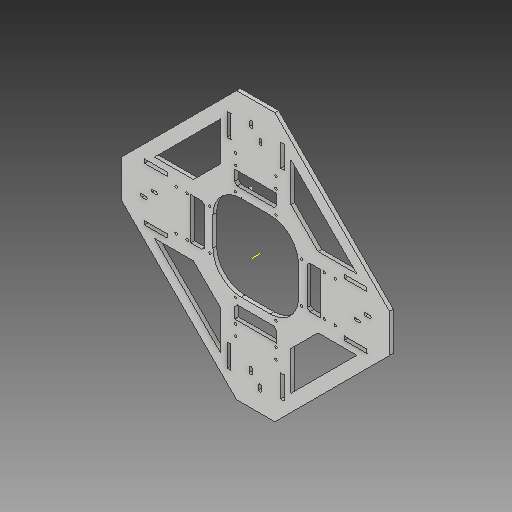
# Autodesk Inventor part: Base Plate
Saved by Autodesk Inventor 2017 (Build 210142000, 142)
## iProperties
Created: 2018-11-23
Part Number: Base Plate
Material: Generic
Document SubType Name: Modeling
Designer: Eric the Great
Density: 1 g/cm^3
Appearance: Default
Author: Eric the Great
Autodesk Inventor part; units mm, degrees
ref_plane "YZ Plane" through (0, 0, 0) normal (1, 0, 0) x (0, 1, 0)
ref_plane "XZ Plane" through (0, 0, 0) normal (0, 1, 0) x (-1, 0, 0)
ref_plane "XY Plane" through (0, 0, 0) normal (0, 0, 1) x (1, 0, 0)
sketch "Sketch1" plane through (0, 0, 0) normal (0, 0, 1) x (1, 0, 0)
  line L0 (79.3342, 54.8946) -> (119.9842, 54.8946)
  line L1 (159.9842, 14.8946) -> (159.9842, -25.7554)
  line L2 (119.9842, -65.7554) -> (79.3342, -65.7554)
  line L3 (39.3342, -25.7554) -> (39.3342, 14.8946)
  line L4 (39.3342, 54.8946) -> (159.9842, -65.7554) construction
  line L5 (159.9842, 54.8946) -> (39.3342, -65.7554) construction
  line L6 (99.6592, 210.0958) -> (315.1854, -5.4304)
  line L7 (315.1854, -5.4304) -> (99.6592, -220.9565)
  line L8 (99.6592, -220.9565) -> (-115.8669, -5.4304)
  line L9 (-115.8669, -5.4304) -> (99.6592, 210.0958)
  line L10 (99.6592, 210.0958) -> (99.6592, -220.9565) construction
  line L11 (315.1854, -5.4304) -> (-115.8669, -5.4304) construction
  arc A0 (39.3342, -25.7554) -> (79.3342, -65.7554) centre (79.3342, -25.7554) ccw
  arc A1 (79.3342, 54.8946) -> (39.3342, 14.8946) centre (79.3342, 14.8946) ccw
  arc A2 (159.9842, 14.8946) -> (119.9842, 54.8946) centre (119.9842, 14.8946) ccw
  arc A3 (119.9842, -65.7554) -> (159.9842, -25.7554) centre (119.9842, -25.7554) ccw
  circle A4 centre (211.7342, 23.0696) radius 1.75 projected
  circle A5 centre (211.7342, -33.9304) radius 1.75 projected
  line L12 (293.5081, -27.1077) -> (293.5081, 16.2469)
  line L13 (195.7506, -101.5218) -> (242.2148, -55.0576)
  line L14 (242.2148, -55.0576) -> (187.4326, -55.0576)
  line L15 (149.2864, -93.2038) -> (149.2864, -147.986)
  line L16 (149.2864, -147.986) -> (195.7506, -101.5218)
  line L17 (168.3595, -74.1307) -> (187.4326, -55.0576)
  line L18 (168.3595, -74.1307) -> (149.2864, -93.2038)
  line L19 (172.0831, 20.9712) -> (172.0831, -31.832)
  line L20 (172.0831, -31.832) -> (176.0974, -34.958)
  line L21 (176.0974, -34.958) -> (191.0974, -34.958)
  line L22 (191.0974, -34.958) -> (191.1331, -34.9121)
  line L23 (191.1331, -34.9121) -> (191.1331, 24.0513)
  line L24 (191.1331, 24.0513) -> (191.0974, 24.0972)
  line L25 (191.0974, 24.0972) -> (176.0974, 24.0972)
  line L26 (176.0974, 24.0972) -> (172.0831, 20.9712)
  line L27 (50.032, -147.986) -> (50.032, -93.2038)
  line L28 (3.5678, -101.5218) -> (50.032, -147.986)
  line L29 (30.9589, -74.1307) -> (50.032, -93.2038)
  line L30 (30.9589, -74.1307) -> (11.8858, -55.0576)
  line L31 (-42.8964, -55.0576) -> (3.5678, -101.5218)
  line L32 (11.8858, -55.0576) -> (-42.8964, -55.0576)
  line L33 (77.9819, -199.2793) -> (121.3365, -199.2793)
  line L34 (126.0608, -77.8543) -> (73.2576, -77.8543)
  line L35 (70.1316, -81.8686) -> (70.1316, -96.8686)
  line L36 (70.1316, -96.8686) -> (70.1775, -96.9043)
  line L37 (129.1868, -81.8686) -> (126.0608, -77.8543)
  line L38 (129.1868, -96.8686) -> (129.1868, -81.8686)
  line L39 (70.1775, -96.9043) -> (129.1409, -96.9043)
  line L40 (129.1409, -96.9043) -> (129.1868, -96.8686)
  line L41 (73.2576, -77.8543) -> (70.1316, -81.8686)
  line L42 (-42.8964, 44.1968) -> (11.8858, 44.1968)
  line L43 (3.5678, 90.661) -> (-42.8964, 44.1968)
  line L44 (30.9589, 63.2699) -> (11.8858, 44.1968)
  line L45 (30.9589, 63.2699) -> (50.032, 82.343)
  line L46 (50.032, 137.1252) -> (3.5678, 90.661)
  line L47 (50.032, 82.343) -> (50.032, 137.1252)
  line L48 (-94.1897, 16.2469) -> (-94.1897, -27.1077)
  line L49 (27.2353, -31.832) -> (27.2353, 20.9712)
  line L50 (23.221, 24.0972) -> (8.221, 24.0972)
  line L51 (8.221, 24.0972) -> (8.1853, 24.0513)
  line L52 (23.221, -34.958) -> (27.2353, -31.832)
  line L53 (8.221, -34.958) -> (23.221, -34.958)
  line L54 (8.1853, 24.0513) -> (8.1853, -34.9121)
  line L55 (8.1853, -34.9121) -> (8.221, -34.958)
  line L56 (27.2353, 20.9712) -> (23.221, 24.0972)
  line L57 (149.2864, 137.1252) -> (149.2864, 82.343)
  line L58 (195.7506, 90.661) -> (149.2864, 137.1252)
  line L59 (168.3595, 63.2699) -> (149.2864, 82.343)
  line L60 (168.3595, 63.2699) -> (187.4326, 44.1968)
  line L61 (242.2148, 44.1968) -> (195.7506, 90.661)
  line L62 (187.4326, 44.1968) -> (242.2148, 44.1968)
  line L63 (121.3365, 188.4185) -> (77.9819, 188.4185)
  line L64 (73.2576, 66.9935) -> (126.0608, 66.9935)
  line L65 (129.1868, 71.0078) -> (129.1868, 86.0078)
  line L66 (129.1868, 86.0078) -> (129.1409, 86.0435)
  line L67 (70.1316, 71.0078) -> (73.2576, 66.9935)
  line L68 (70.1316, 86.0078) -> (70.1316, 71.0078)
  line L69 (129.1409, 86.0435) -> (70.1775, 86.0435)
  line L70 (70.1775, 86.0435) -> (70.1316, 86.0078)
  line L71 (126.0608, 66.9935) -> (129.1868, 71.0078)
  circle A6 centre (128.1592, -101.9862) radius 1.75 projected
  circle A7 centre (71.1592, -101.9862) radius 1.75 projected
  circle A8 centre (71.1592, -117.5054) radius 1.75 projected
  circle A9 centre (128.1592, -117.5054) radius 1.75 projected
  line L72 (95.4092, -166.1418) -> (95.4092, -160.1418) projected
  arc A10 (95.4092, -160.1418) -> (91.4092, -160.1418) centre (93.4092, -160.1418) ccw projected
  arc A11 (91.4092, -166.1418) -> (95.4092, -166.1418) centre (93.4092, -166.1418) ccw projected
  line L73 (103.9092, -145.6418) -> (103.9092, -151.6418) projected
  arc A12 (103.9092, -151.6418) -> (107.9092, -151.6418) centre (105.9092, -151.6418) ccw projected
  line L74 (107.9092, -151.6418) -> (107.9092, -145.6418) projected
  arc A13 (107.9092, -145.6418) -> (103.9092, -145.6418) centre (105.9092, -145.6418) ccw projected
  line L75 (90.8763, -145.4109) -> (90.8763, -151.4109) projected
  line L76 (94.8763, -151.4109) -> (94.8763, -145.4109) projected
  arc A14 (90.8763, -151.4109) -> (94.8763, -151.4109) centre (92.8763, -151.4109) ccw projected
  arc A15 (94.8763, -145.4109) -> (90.8763, -145.4109) centre (92.8763, -145.4109) ccw projected
  arc A16 (107.9092, -160.1418) -> (103.9092, -160.1418) centre (105.9092, -160.1418) ccw projected
  line L77 (103.9092, -160.1418) -> (103.9092, -166.1418) projected
  arc A17 (103.9092, -166.1418) -> (107.9092, -166.1418) centre (105.9092, -166.1418) ccw projected
  line L78 (107.9092, -166.1418) -> (107.9092, -160.1418) projected
  circle A18 centre (128.1592, -70.0054) radius 1.75 projected
  circle A19 centre (71.1592, -70.0054) radius 1.75 projected
  line L79 (139.9592, -130.3297) -> (134.6592, -130.3297) projected
  line L80 (139.9592, -162.0797) -> (134.6592, -162.0797) projected
  line L81 (139.9592, -162.0797) -> (139.9592, -130.3297) projected
  line L82 (134.6592, -130.3297) -> (134.6592, -162.0797) projected
  line L83 (64.6592, -130.3297) -> (59.3592, -130.3297) projected
  line L84 (59.3592, -130.3297) -> (59.3592, -162.0797) projected
  line L85 (64.6592, -162.0797) -> (64.6592, -130.3297) projected
  line L86 (64.6592, -162.0797) -> (59.3592, -162.0797) projected
  line L87 (139.9592, -130.3297) -> (134.6592, -130.3297)
  line L88 (134.6592, -130.3297) -> (134.6592, -162.0797)
  line L89 (134.6592, -162.0797) -> (139.9592, -162.0797)
  line L90 (139.9592, -162.0797) -> (139.9592, -130.3297)
  line L91 (64.6592, -130.3297) -> (59.3592, -130.3297)
  line L92 (59.3592, -130.3297) -> (59.3592, -162.0797)
  line L93 (59.3592, -162.0797) -> (64.6592, -162.0797)
  line L94 (64.6592, -162.0797) -> (64.6592, -130.3297)
  circle A20 centre (128.1592, -70.0054) radius 1.75
  circle A21 centre (71.1592, -70.0054) radius 1.75
  circle A22 centre (71.1592, -101.9862) radius 1.75
  circle A23 centre (71.1592, -117.5054) radius 1.75
  circle A24 centre (128.1592, -117.5054) radius 1.75
  line L95 (92.8763, -151.4109) -> (92.8763, -145.4109) construction
  line L96 (94.4027, -151.4109) -> (94.4027, -145.4109)
  line L97 (91.35, -145.4109) -> (91.35, -151.4109)
  arc A25 (91.35, -151.4109) -> (94.4027, -151.4109) centre (92.8763, -151.4109) ccw
  arc A26 (94.4027, -145.4109) -> (91.35, -145.4109) centre (92.8763, -145.4109) ccw
  line L98 (105.9092, -166.1418) -> (105.9092, -160.1418) construction
  line L99 (107.9092, -166.1418) -> (107.9092, -160.1418)
  line L100 (103.9092, -160.1418) -> (103.9092, -166.1418)
  arc A27 (103.9092, -166.1418) -> (107.9092, -166.1418) centre (105.9092, -166.1418) ccw
  arc A28 (107.9092, -160.1418) -> (103.9092, -160.1418) centre (105.9092, -160.1418) ccw
  circle A29 centre (128.1592, -101.9862) radius 1.75
  circle A30 centre (164.2342, 23.0696) radius 1.75
  circle A31 centre (164.2342, -33.9304) radius 1.75
  circle A32 centre (196.215, 23.0696) radius 1.75
  circle A33 centre (211.7342, 23.0696) radius 1.75
  circle A34 centre (196.215, -33.9304) radius 1.75
  circle A35 centre (211.7342, -33.9304) radius 1.75
  circle A36 centre (71.1592, 59.1446) radius 1.75
  circle A37 centre (128.1592, 59.1446) radius 1.75
  circle A38 centre (71.1592, 91.1254) radius 1.75
  circle A39 centre (71.1592, 106.6446) radius 1.75
  circle A40 centre (128.1592, 91.1254) radius 1.75
  circle A41 centre (128.1592, 106.6446) radius 1.75
  circle A42 centre (35.0842, -33.9304) radius 1.75
  circle A43 centre (35.0842, 23.0696) radius 1.75
  circle A44 centre (3.1034, -33.9304) radius 1.75
  circle A45 centre (-12.4158, -33.9304) radius 1.75
  circle A46 centre (3.1034, 23.0696) radius 1.75
  circle A47 centre (-12.4158, 23.0696) radius 1.75
  line L101 (256.3086, -45.7304) -> (256.3086, -40.4304)
  line L102 (256.3086, -40.4304) -> (224.5586, -40.4304)
  line L103 (224.5586, -40.4304) -> (224.5586, -45.7304)
  line L104 (224.5586, -45.7304) -> (256.3086, -45.7304)
  line L105 (224.5586, 34.8696) -> (224.5586, 29.5696)
  line L106 (256.3086, 29.5696) -> (256.3086, 34.8696)
  line L107 (224.5586, 29.5696) -> (256.3086, 29.5696)
  line L108 (256.3086, 34.8696) -> (224.5586, 34.8696)
  line L109 (139.9592, 151.219) -> (134.6592, 151.219)
  line L110 (134.6592, 151.219) -> (134.6592, 119.469)
  line L111 (134.6592, 119.469) -> (139.9592, 119.469)
  line L112 (139.9592, 119.469) -> (139.9592, 151.219)
  line L113 (59.3592, 119.469) -> (64.6592, 119.469)
  line L114 (64.6592, 151.219) -> (59.3592, 151.219)
  line L115 (64.6592, 119.469) -> (64.6592, 151.219)
  line L116 (59.3592, 151.219) -> (59.3592, 119.469)
  line L117 (-56.9901, 34.8696) -> (-56.9901, 29.5696)
  line L118 (-56.9901, 29.5696) -> (-25.2401, 29.5696)
  line L119 (-25.2401, 29.5696) -> (-25.2401, 34.8696)
  line L120 (-25.2401, 34.8696) -> (-56.9901, 34.8696)
  line L121 (-25.2401, -45.7304) -> (-25.2401, -40.4304)
  line L122 (-56.9901, -40.4304) -> (-56.9901, -45.7304)
  line L123 (-25.2401, -40.4304) -> (-56.9901, -40.4304)
  line L124 (-56.9901, -45.7304) -> (-25.2401, -45.7304)
  line L125 (254.3706, -1.1804) -> (260.3706, -1.1804)
  line L126 (260.3706, 0.8196) -> (254.3706, 0.8196) construction
  line L127 (260.3706, 2.8196) -> (254.3706, 2.8196)
  arc A48 (254.3706, 2.8196) -> (254.3706, -1.1804) centre (254.3706, 0.8196) ccw
  arc A49 (260.3706, -1.1804) -> (260.3706, 2.8196) centre (260.3706, 0.8196) ccw
  arc A50 (245.6397, -13.7396) -> (245.6397, -10.6869) centre (245.6397, -12.2133) ccw
  line L128 (245.6397, -10.6869) -> (239.6397, -10.6869)
  line L129 (245.6397, -12.2133) -> (239.6397, -12.2133) construction
  line L130 (239.6397, -13.7396) -> (245.6397, -13.7396)
  arc A51 (239.6397, -10.6869) -> (239.6397, -13.7396) centre (239.6397, -12.2133) ccw
  line L131 (95.4092, 149.281) -> (95.4092, 155.281)
  line L132 (93.4092, 155.281) -> (93.4092, 149.281) construction
  line L133 (91.4092, 155.281) -> (91.4092, 149.281)
  arc A52 (91.4092, 149.281) -> (95.4092, 149.281) centre (93.4092, 149.281) ccw
  arc A53 (95.4092, 155.281) -> (91.4092, 155.281) centre (93.4092, 155.281) ccw
  arc A54 (107.9684, 140.5501) -> (104.9157, 140.5501) centre (106.4421, 140.5501) ccw
  line L134 (104.9157, 140.5501) -> (104.9157, 134.5501)
  line L135 (106.4421, 140.5501) -> (106.4421, 134.5501) construction
  line L136 (107.9684, 134.5501) -> (107.9684, 140.5501)
  arc A55 (104.9157, 134.5501) -> (107.9684, 134.5501) centre (106.4421, 134.5501) ccw
  line L137 (-55.0522, -9.6804) -> (-61.0522, -9.6804)
  line L138 (-61.0522, -11.6804) -> (-55.0522, -11.6804) construction
  line L139 (-61.0522, -13.6804) -> (-55.0522, -13.6804)
  arc A56 (-55.0522, -13.6804) -> (-55.0522, -9.6804) centre (-55.0522, -11.6804) ccw
  arc A57 (-61.0522, -9.6804) -> (-61.0522, -13.6804) centre (-61.0522, -11.6804) ccw
  arc A58 (-46.3213, 2.8788) -> (-46.3213, -0.1739) centre (-46.3213, 1.3525) ccw
  line L140 (-46.3213, -0.1739) -> (-40.3213, -0.1739)
  line L141 (-46.3213, 1.3525) -> (-40.3213, 1.3525) construction
  line L142 (-40.3213, 2.8788) -> (-46.3213, 2.8788)
  arc A59 (-40.3213, -0.1739) -> (-40.3213, 2.8788) centre (-40.3213, 1.3525) ccw
  point P0 (0, 0)
  point P1 (99.6592, -5.4304)
  point P2 (99.6592, -5.4304)
  point P3 (99.6592, -5.4304)
  point P4 (99.6592, -5.4304)
  point P5 (244.9497, 7.0696)
  point P6 (244.9497, -17.9304)
  point P7 (270.9497, 7.0696)
  point P8 (270.9497, -17.9304)
  point P9 (215.9842, -37.9304)
  point P10 (215.9842, 27.0696)
  point P11 (207.4842, 27.0696)
  point P12 (207.4842, -37.9304)
  point P13 (39.3342, -65.7554)
  point P14 (39.3342, -25.7554)
  point P15 (112.1592, -150.7209)
  point P16 (87.1592, -150.7209)
  point P17 (112.1592, -176.7209)
  point P18 (87.1592, -176.7209)
  point P19 (128.1592, -117.5054)
  point P20 (71.1592, -117.5054)
  point P21 (67.1592, -121.7554)
  point P22 (132.1592, -113.2554)
  point P23 (67.1592, -113.2554)
  point P24 (132.1592, -121.7554)
  point P25 (39.3342, 54.8946)
  point P26 (79.3342, 54.8946)
  point P27 (-45.6313, -17.9304)
  point P28 (-45.6313, 7.0696)
  point P29 (-71.6313, -17.9304)
  point P30 (-71.6313, 7.0696)
  point P31 (-12.4158, -33.9304)
  point P32 (-12.4158, 23.0696)
  point P33 (-16.6658, 27.0696)
  point P34 (-8.1658, -37.9304)
  point P35 (-8.1658, 27.0696)
  point P36 (-16.6658, -37.9304)
  point P37 (159.9842, 54.8946)
  point P38 (159.9842, 14.8946)
  point P39 (87.1592, 139.8601)
  point P40 (112.1592, 139.8601)
  point P41 (87.1592, 165.8601)
  point P42 (112.1592, 165.8601)
  point P43 (71.1592, 106.6446)
  point P44 (128.1592, 106.6446)
  point P45 (132.1592, 110.8946)
  point P46 (67.1592, 102.3946)
  point P47 (132.1592, 102.3946)
  point P48 (67.1592, 110.8946)
  point P49 (92.8763, -148.4109)
  point P50 (105.9092, -163.1418)
  point P51 (207.4842, 27.0696)
  point P52 (211.7342, 23.0696)
  point P53 (211.7342, -33.9304)
  point P54 (211.7342, -33.9304)
  point P55 (207.4842, -37.9304)
  point P56 (67.1592, 102.3946)
  point P57 (71.1592, 106.6446)
  point P58 (128.1592, 106.6446)
  point P59 (132.1592, 102.3946)
  point P60 (35.0842, -33.9304)
  point P61 (-8.1658, -37.9304)
  point P62 (-12.4158, -33.9304)
  point P63 (-12.4158, 23.0696)
  point P64 (-8.1658, 27.0696)
  point P65 (256.3086, -40.4304)
  point P66 (134.6592, 151.219)
  point P67 (-56.9901, 29.5696)
  point P68 (257.3706, 0.8196)
  point P69 (260.3706, -1.1804)
  point P70 (245.6397, -10.2133)
  point P71 (245.6397, -14.2133)
  point P72 (239.6397, -10.2133)
  point P73 (239.6397, -14.2133)
  point P74 (242.6397, -12.2133)
  point P75 (93.4092, 152.281)
  point P76 (95.4092, 155.281)
  point P77 (104.4421, 140.5501)
  point P78 (108.4421, 140.5501)
  point P79 (104.4421, 134.5501)
  point P80 (108.4421, 134.5501)
  point P81 (106.4421, 137.5501)
  point P82 (-58.0522, -11.6804)
  point P83 (-61.0522, -9.6804)
  point P84 (-46.3213, -0.6475)
  point P85 (-46.3213, 3.3525)
  point P86 (-40.3213, -0.6475)
  point P87 (-40.3213, 3.3525)
  point P88 (-43.3213, 1.3525)
  dimension "d0" = 120.65
  dimension "d1" = 120.65
  dimension "d11" = 304.8
  dimension "d12" = 304.8
  dimension "d13" = 40
  dimension "d14" = 15
  dimension "d17" = 360
  dimension "d22" = 19.05
  dimension "d24" = 31.75
  dimension "d25" = 5.3
  dimension "d28" = 360
  dimension "d32" = 360
  dimension "d36" = 360
  constraints: 272 end point, 44 centre point, 40 point on circle, 24 coincident, 16 tangent, 14 parallel, 11 point on line, 9 equal radius, 9 midpoint, 9 perpendicular, 6 equal length, 3 horizontal, 2 collinear, 2 vertical, 474 other
  measures "d0" distance of L5.start L4.end
  measures "d1" distance of L4.end L5.end
  measures "d11" distance of L6.end L7.end
  measures "d12" distance of L7.end L8.end
  measures "d13" radius of A0
  measures "d14" distance of L20.end L21.end
  measures "d22" distance between parallel lines of L49 L54
  measures "d24" distance of L85.start L83.start
  measures "d25" distance of L83.start L83.end
extrude "Extrusion1" add sketch "Sketch1" along normal mid plane 5.3 contours L6 L63 L9 | L6 L12 L7 L33 L8 L48 L9 L63 | L6 L7 L12 | L48 L8 L9 | L7 L8 L33 | A13 L74 A12 L73
chamfer "Chamfer1" distance 38.1 angle 45 4 edges at (-115.8669, -5.4304, 0) (99.6592, 210.0958, 0) (315.1854, -5.4304, 0) (99.6592, -220.9565, 0)
ref_plane "Work Plane1" through (99.6592, -25.7554, -2.65) normal (1, 0, 0) x (0, 0, -1)
ref_plane "Work Plane2" through (79.3342, -5.4304, -2.65) normal (0, -1, 0) x (1, 0, 0)
body "Solid1"
